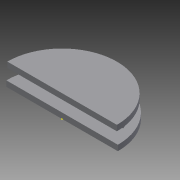
# Autodesk Inventor part: Top Holder
Saved by Autodesk Inventor 2015 (Build 190159000, 159)
## iProperties
Created: 2016-05-27
Part Number: Top Holder
Material: Generic
Document SubType Name: Modeling
Designer: Toby
Density: 1 g/cm^3
Appearance: Default
Author: Toby
Autodesk Inventor part; units mm, degrees
ref_plane "YZ Plane" through (0, 0, 0) normal (1, 0, 0) x (0, 1, 0)
ref_plane "XZ Plane" through (0, 0, 0) normal (0, 1, 0) x (-1, 0, 0)
ref_plane "XY Plane" through (0, 0, 0) normal (0, 0, 1) x (1, 0, 0)
sketch "Sketch1" plane through (0, 0, 0) normal (0, 0, 1) x (1, 0, 0)
  circle A0 centre (0, 0) radius 10
  dimension "d0" = 20
  constraints: 1 centre point, 1 coincident
  measures "d0" diameter of A0
extrude "Extrusion1" add sketch "Sketch1" along normal blind 1
sketch "Sketch2" plane through (0, 0, 1) normal (0, 0, 1) x (1, 0, 0)
  circle A0 centre (0, 0) radius 8.5
  dimension "d3" = 17
  constraints: 1 centre point, 1 coincident
  measures "d3" diameter of A0
extrude "Extrusion2" add sketch "Sketch2" along normal blind 2
sketch "Sketch3" plane through (0, 0, 3) normal (0, 0, 1) x (1, 0, 0)
  circle A0 centre (0, 0) radius 9.8227
  constraints: 1 centre point, 1 coincident
extrude "Extrusion3" add sketch "Sketch3" along normal blind 1
sketch "Sketch4" plane through (0, 0, 4) normal (0, 0, 1) x (1, 0, 0)
  circle A0 centre (0, 0) radius 4.5
  line L0 (-3.25, 1.75) -> (3.25, 1.75)
  line L1 (3.25, 1.75) -> (3.25, -1.75)
  line L2 (3.25, -1.75) -> (-3.25, -1.75)
  line L3 (-3.25, -1.75) -> (-3.25, 1.75)
  dimension "d8" = 9
  dimension "d9" = 3.5
  dimension "d10" = 6.5
  dimension "d11" = 1.75
  dimension "d12" = 3.25
  constraints: 8 end point, 2 parallel, 1 centre point, 1 coincident, 1 horizontal, 1 perpendicular
  measures "d8" diameter of A0
  measures "d9" distance of L2.end L0.start
  measures "d10" distance of L0.start L0.end
  measures "d11" distance from line of point (0, 0) L0
  measures "d12" distance from line of point (0, 0) L3
extrude "Extrusion4" add sketch "Sketch4" along normal blind 7
sketch "Sketch5" plane through (0, 0, 0) normal (0, 0, -1) x (-1, 0, 0)
  point P0 (0, 0)
sketch "Sketch6" plane through (0, 0, 11) normal (0, 0, 1) x (1, 0, 0)
  circle A0 centre (0, 0) radius 4.5
  constraints: 1 centre point, 1 coincident
extrude "Extrusion5" cut sketch "Sketch6" against normal blind 7
sketch "Sketch7" plane through (0, 0, 4) normal (0, 0, 1) x (1, 0, 0)
  line L0 (-13.328, 0) -> (12.5041, 0)
  line L1 (12.5041, 0) -> (12.5041, -10.2387)
  line L2 (12.5041, -10.2387) -> (-13.328, -10.2387)
  line L3 (-13.328, -10.2387) -> (-13.328, 0)
  point P0 (0, 0)
  constraints: 8 end point, 2 parallel, 1 horizontal, 1 perpendicular
extrude "Extrusion6" cut sketch "Sketch7" against normal blind 10
sketch "Sketch8" plane through (-9.8227, 0, 4) normal (0, -1, 0) x (1, 0, 0)
  line L0 (19.8227, -3) -> (-0.1773, -3) projected
  line L1 (1.3199, -0.999) -> (18.3844, -0.999)
  line L2 (18.3844, -0.999) -> (18.3844, -3)
  line L3 (18.3844, -3) -> (1.3199, -3)
  line L4 (1.3199, -3) -> (1.3199, -0.999)
  point P0 (9.8227, -4)
  constraints: 8 end point, 2 parallel, 1 horizontal, 1 perpendicular, 1 point on line
extrude "Extrusion7" cut sketch "Sketch8" against normal blind 3
body "Solid1"
